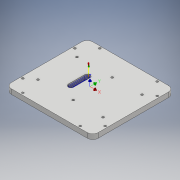
# Autodesk Inventor part: Parte4
Saved by Autodesk Inventor 2017 (Build 210142000, 142)
## iProperties
Part Number: Parte4
Material: Generico
Document SubType Name: Modeling
Designer: Federico
Density: 1 g/cm^3
Appearance: Default
Author: Federico
Autodesk Inventor part; units mm, degrees
ref_plane "YZ Plane" through (0, 0, 0) normal (1, 0, 0) x (0, 1, 0)
ref_plane "XZ Plane" through (0, 0, 0) normal (0, 1, 0) x (-1, 0, 0)
ref_plane "XY Plane" through (0, 0, 0) normal (0, 0, 1) x (1, 0, 0)
sketch "Schizzo1" plane through (0, 0, 0) normal (0, 0, 1) x (1, 0, 0)
  line L0 (75, -65) -> (75, 65)
  line L1 (65, 75) -> (-75, 75)
  line L2 (-85, 65) -> (-85, -65)
  line L3 (-75, -75) -> (65, -75)
  circle A0 centre (0, -36) radius 2
  circle A1 centre (0, 36) radius 2
  circle A2 centre (55, -36) radius 2
  circle A3 centre (55, 36) radius 2
  circle A4 centre (-65, -36) radius 2
  circle A5 centre (-65, 36) radius 2
  arc A6 (-85, -65) -> (-75, -75) centre (-75, -65) ccw
  arc A7 (-75, 75) -> (-85, 65) centre (-75, 65) ccw
  arc A8 (75, 65) -> (65, 75) centre (65, 65) ccw
  arc A9 (65, -75) -> (75, -65) centre (65, -65) ccw
  line L4 (-25, -20) -> (-25, -20)
  line L5 (-20, -15) -> (-20, 15)
  line L6 (-25, 20) -> (-25, 20)
  line L7 (-30, 15) -> (-30, -15)
  arc A10 (-30, -15) -> (-25, -20) centre (-25, -15) ccw
  arc A11 (-25, -20) -> (-20, -15) centre (-25, -15) ccw
  arc A12 (-20, 15) -> (-25, 20) centre (-25, 15) ccw
  arc A13 (-25, 20) -> (-30, 15) centre (-25, 15) ccw
  line L8 (75, -65) -> (75, 65)
  line L9 (65, 75) -> (-75, 75)
  line L10 (-85, 65) -> (-85, -65)
  line L11 (-75, -75) -> (65, -75)
  arc A14 (-85, -65) -> (-75, -75) centre (-75, -65) ccw
  arc A15 (-75, 75) -> (-85, 65) centre (-75, 65) ccw
  arc A16 (75, 65) -> (65, 75) centre (65, 65) ccw
  arc A17 (65, -75) -> (75, -65) centre (65, -65) ccw
  circle A18 centre (-81, 48) radius 2
  circle A19 centre (-81, -48) radius 2
  circle A20 centre (71, 48) radius 2
  circle A21 centre (71, -48) radius 2
  circle A22 centre (-58, -71) radius 2
  circle A23 centre (-58, 71) radius 2
  circle A24 centre (48, 71) radius 2
  circle A25 centre (48, -71) radius 2
  point P0 (0, 0)
  point P1 (0, 0)
  point P2 (0, 0)
  point P3 (-25, 0)
  dimension "d0" = 4
  dimension "d1" = 4
  dimension "d2" = 4
  dimension "d3" = 4
  dimension "d4" = 4
  dimension "d5" = 4
  dimension "d6" = 10
  dimension "d7" = 5
  dimension "d8" = 10
  dimension "d9" = 4
  dimension "d10" = 4
  dimension "d11" = 4
  dimension "d12" = 4
  dimension "d13" = 4
  dimension "d14" = 4
  dimension "d15" = 4
  dimension "d16" = 4
  constraints: 26 centre point, 24 end point, 24 point on circle, 24 tangent, 9 equal radius, 3 perpendicular, 2 parallel, 1 horizontal
  measures "d0" diameter of A0
  measures "d1" diameter of A1
  measures "d2" diameter of A2
  measures "d3" diameter of A3
  measures "d4" diameter of A4
  measures "d5" diameter of A5
  measures "d6" radius of A6
  measures "d7" radius of A10
  measures "d8" radius of A14
  measures "d9" diameter of A18
  measures "d10" diameter of A19
  measures "d11" diameter of A20
  measures "d12" diameter of A21
  measures "d13" diameter of A22
  measures "d14" diameter of A23
  measures "d15" diameter of A24
  measures "d16" diameter of A25
extrude "Estrusione1" add sketch "Schizzo1" along normal blind 9
